Autodesk Fusion 360 part; units mm, degrees
(part 2 of 2)
  constraint coincident L135 L316.end
  constraint coincident L135 L317.end
  constraint coincident L135 L321.end
  constraint perpendicular L135 L321
  constraint coincident L135 L322.end
  constraint perpendicular L135 L322
  measures "d208" distance of L26.start L13.start
  measures "d209" distance of L9.start L13.start
  measures "d210" distance of L2.start L2.end
  measures "d211" distance of L1.start L2.end
  measures "d212" distance of L0.start L4.start
  measures "d213" distance of L23.start L21.end
  measures "d214" distance of L23.start L22.end
  measures "d217" distance of L8.start L54.end
  measures "d218" distance of L53.start L54.end
  measures "d234" distance of L40.start L40.end
  measures "d254" diameter of A0
  measures "d255" diameter of A2
  measures "d256" diameter of A12
  measures "d257" distance of L0.end L0.start
  measures "d265" distance of L10.start A1.centre
  measures "d266" distance of L10.start L10.end
  measures "d267" diameter of A3
  measures "d268" diameter of A1
  measures "d269" distance of L9.end L18.start
  measures "d270" distance of L9.end L17.start
  measures "d271" distance of L9.start L24.start
  measures "d272" distance of L9.start L11.start
  measures "d273" distance of L17.start L9.end
  measures "d274" distance of L11.start L28.start
  measures "d275" distance of L11.start L9.start
  measures "d276" distance of L38.start L18.end
  measures "d277" distance of L43.end L18.end
  measures "d278" diameter of A6
  measures "d279" distance of L35.start L24.end
  measures "d280" distance of L39.end L24.end
  measures "d281" diameter of A11
  measures "d300" distance of L22.start L63.end
  measures "d301" distance of L23.start L67.end
  measures "d303" distance of L71.start L71.end
  measures "d304" distance of L72.start L72.end
  measures "d305" distance of L55.end L73.end
  measures "d306" distance of L55.start L77.end
  measures "d307" distance of L57.end L84.end
  measures "d308" distance of L86.start L86.end
  measures "d310" distance of L5.start L91.end
  measures "d311" distance of L93.start L93.end
  measures "d312" distance of L94.start L94.end
  measures "d313" distance of L95.start L95.end
  measures "d314" distance of L96.start L96.end
  measures "d315" diameter of A13
  measures "d316" diameter of A14
  measures "d319" distance of L110.start L110.end
  measures "d320" distance of L110.start L111.end
  measures "d325" distance of L121.start L121.end
  measures "d326" distance of L121.start L122.end
  measures "d327" distance of L125.start L125.end
  measures "d328" distance of L125.start L129.end
  measures "d329" distance of L55.start L135.end
  measures "d334" distance of L0.end L139.end
  measures "d335" distance of L5.start L141.end
  measures "d336" distance of L4.start L145.end
  measures "d338" distance of L149.start L149.end
  measures "d339" distance of L149.start L150.end
  measures "d342" distance of L152.start L152.end
  measures "d343" distance of L152.start L153.end
  measures "d344" distance of L159.start L159.end
  measures "d345" distance of L159.start L160.end
  measures "d346" diameter of A15
  measures "d347" distance of L167.start L167.end
  measures "d348" distance of L168.start L168.end
  measures "d349" distance of L173.start L173.end
  measures "d350" distance of L174.start L174.end
  measures "d354" distance of L182.start L182.end
  measures "d356" distance of L188.start L188.end
  measures "d357" distance of L188.start L189.end
  measures "d358" distance of L194.start L194.end
  measures "d371" distance of L22.start L205.end
  measures "d372" distance of L22.end L209.end
  measures "d375" distance of L1.start L213.end
  measures "d376" distance of L2.end L217.end
  measures "d377" distance of L221.start L221.end
  measures "d378" distance of L222.start L222.end
  measures "d379" distance of L226.start L226.end
  measures "d380" distance of L1.end L231.end
  measures "d381" distance of L233.start L233.end
  measures "d382" distance of L233.start L236.end
  measures "d383" distance of L242.start L242.end
  measures "d384" distance of L242.start L243.end
  measures "d385" distance of L244.start L244.end
  measures "d386" distance of L244.start L245.end
  measures "d387" distance of L251.start L251.end
  measures "d388" distance of L251.start L252.end
  measures "d391" distance of L260.start L260.end
  measures "d392" distance of L260.start L262.end
  measures "d393" distance of L260.start L266.end
  measures "d396" distance of L270.start L270.end
  measures "d397" distance of L270.start L272.end
  measures "d398" distance of L270.start L270.end
  measures "d399" distance of L270.start L276.end
  measures "d400" diameter of A16
  measures "d401" diameter of A17
  measures "d404" distance of L13.start L290.end
  measures "d405" distance of L24.end L298.end
  measures "d411" distance of A8.centre L307.end
  measures "d412" distance of A4.centre L308.end
extrude "Extrude13" add sketch "v0.2" along normal blind 4 contours A0 L157 L164 | A0 L151 L157 L158 L164 A15 | A0 L157 L164 | A0 L157 L164 A15 | L158 L160 L164 A15 | L151 L152 L157 A15 | L5 L89 L158 L160 L161 | L0 L137 L149 L158 A15 | L0 L137 L149 L158 L159 L163 A15 | L5 L89 L151 L152 L154 | L0 L137 L150 L151 L153 L156 A15 | L0 L137 L150 L151 A15 | L146 L158 L159 L162 | L5 L16 L89 L90 L91 L145 | L0 L137 L149 L150 A15 | L0 L137 L138 L139 L140 L143 L147 L149 L150 A15 L233 L236 | L142 L151 L153 L155 | L5 L16 L89 L91 L92 L141 | L0 L4 L5 L89 L137 L145 L146 L147 L148 | L0 L5 L6 L89 L137 L141 L142 L143 L144 | L0 L137 L142 L150 L155 L156 | L31 L90 L91 L94 L99 L105 | L21 L91 L92 L95 L101 L116 | L31 L94 L96 L98 L104 L105 | L91 L166 L174 L176 | L23 L91 L165 L171 | L21 L93 L95 L97 L116 L117 | L23 L31 L67 L96 L102 L211 | L94 L99 L105 | L94 L98 A14 L105 | L23 L99 L166 L178 | L15 L23 L166 L175 | L23 L166 L174 L175 | L23 L165 L167 L171 | L23 L101 L165 L172 | L21 L23 L65 L93 L100 L207 | L95 A13 L116 | L95 L101 A13 L116 | L22 L23 L51 L67 L68 L69 L70 L209 L211 L212 | L23 L98 L102 L104 L108 | L98 A14 | L98 A14 L104 L105 | L15 L23 L166 L178 | L15 L22 L166 L175 L203 | L23 L165 L168 L172 | L10 L165 L167 L170 | L22 L23 L25 L63 L64 L65 L66 L205 L207 L208 | L23 L97 L100 L117 L119 | L95 L97 A13 | L95 L101 A13 | L97 A13 L116 L117 | L23 L68 L102 L210 L211 | L22 L62 L69 L72 L81 L209 | L98 A14 L109 | L23 A12 L98 A14 L107 | L10 L22 L165 L170 | L15 L166 L173 L178 | L10 L165 L168 L169 | L22 L61 L63 L86 L205 | L97 A13 L117 | A2 L23 L97 L101 A13 L118 | L101 A13 L120 | L23 L102 L210 | L22 L68 L81 L209 L210 | L62 L71 L72 L179 L180 | L23 A14 L104 | L23 L104 L108 | L23 A12 A14 L107 | L15 L178 L184 | L10 L22 L165 L169 | L22 L165 L170 L201 | L15 L22 L178 L181 L184 | L22 L166 L173 L177 | L22 L84 L166 L177 L204 | L22 L64 L87 L205 L206 | L22 L61 L84 L85 L86 L185 L186 | L23 A13 L117 | L23 L117 L119 | A2 L23 A13 L118 | L22 L81 L210 | L62 L71 L83 L84 L88 L179 | L22 L81 L112 L113 L180 | L23 A14 L104 L108 | L23 A12 A14 L107 | L15 L23 A12 A14 L107 | L10 L169 L193 | L10 L22 L169 L187 L193 | L22 L84 L165 L169 | L22 L177 L178 L181 L196 | L22 L177 L196 | L57 L75 L79 L82 L83 L84 L85 L127 L131 | A2 L10 L23 A13 L118 | L22 L86 L87 L206 | L55 L57 L58 L77 L78 L79 L80 L82 L133 | L22 L86 L185 | A2 L23 A13 L118 | L23 A13 L117 L119 | L55 L56 L57 L73 L74 L75 L76 L82 L133 | L88 L179 L181 L194 L195 | L15 A14 L199 | L15 A14 L103 L111 L199 | L22 L181 L182 L184 | L22 L169 L187 L192 | L22 L169 L192 | L22 L181 L194 L196 | L10 A13 L197 | L10 A13 L114 L121 L197 | L55 L73 L77 L125 L129 L133 L134 L135 L136 | L22 L103 L110 L111 L112 L113 | L179 L181 L182 L183 | L15 A14 L200 | L15 A14 | L22 L187 L189 L193 | L22 L187 L188 L192 | L10 A13 | L22 L114 L121 L122 L123 L124 | L55 L57 L82 L128 L129 L130 L131 L132 L133 | L22 L123 L124 L185 | L10 A13 L198 | L15 A14 L103 L110 L200 | L55 L57 L82 L125 L126 L127 L128 L132 L133 | L186 L187 L189 L190 | L186 L187 L188 L191 | L10 A13 L114 L122 L198 makes body 1
extrude "Extrude14" add sketch "v0.2" along normal blind 4 separate body contours L98 A14 L104 makes body 2
extrude "Extrude15" add sketch "v0.2" along normal blind 4 contours L15 L22 L166 L175 L203 bodies 1
combine "Combine1" operation add target body 1 tool bodies 2
extrude "Extrude16" add sketch "v0.2" along normal blind 4 contours L22 L166 L175 L201 L202 L203 L204 bodies 1
extrude "Extrude17" cut sketch "v0.2" along normal blind 4 contours L22 L170 L175 L202 bodies 1
extrude "Extrude18" add sketch "v0.2" along normal blind 4 contours L23 L64 L100 L206 L207 | L23 L100 L119 | L23 L100 L206 bodies 1
extrude "Extrude19" add sketch "v0.2" along normal blind 4 contours L15 L68 L102 L210 | L10 L64 L100 L206 | L15 L68 L81 L210 | L10 L64 L87 L206 bodies 1
copy_body "CopyPasteBodies1" bodies 1 makes body 3
extrude "Extrude20" add sketch "v0.2" along normal blind 4 contours L7 L138 L139 L222 L224 | L3 L139 L140 L226 L228 | L7 L221 L222 L223 | L3 L217 L218 L226 L227 | L7 L213 L214 L221 L225 | L2 L217 L218 L220 L239 | L1 L213 L214 L216 L239 | L224 L246 L247 L256 | L139 L233 L234 L236 L237 L258 | L2 L218 L220 L231 L239 | L228 L248 L249 L258 | L1 L214 L216 L231 L239 L250 L251 L252 | L214 L246 L256 L257 | L246 L247 L256 L257 | L234 L247 L256 L257 L258 L259 | L234 L237 L258 L259 | L2 L14 L218 L219 L220 L229 L230 L231 | L218 L249 L258 L259 | L248 L249 L258 L259 | L237 L248 L258 L259 | L1 L14 L214 L215 L216 L229 L231 L232 | L239 L246 L247 L255 L257 | L234 L262 L268 | L234 L237 L239 L259 L263 L273 | L9 L14 L19 L37 L44 L47 L214 L218 L229 L231 L235 L238 L240 L241 L242 L243 L244 L245 L292 | L218 L249 L253 L254 | L239 L248 L249 L259 | L239 L248 L249 L254 | L237 L272 L278 | L214 L231 L240 L246 L250 L253 | L214 L246 L250 L251 L252 L253 L254 | L239 L246 L247 L254 L255 | L234 L239 L260 L261 L262 L263 L264 A16 | L231 L241 L242 L243 L248 L249 L253 | L248 L249 L253 L254 | L237 L239 L270 L271 L272 L273 L274 A17 | L231 L240 L244 L245 L246 L247 L253 | L246 L247 L253 L254 | L234 L239 L260 L264 L265 L266 L267 A16 | L234 L237 L239 L254 L267 L277 | L234 L247 L253 L254 | L237 L248 L253 L254 | L237 L239 L270 L274 L275 L276 L277 A17 | L234 L266 L269 | L234 L237 L253 L254 | L237 L276 L279 | L231 L234 L235 L237 L238 L253 bodies 3
extrude "Extrude21" add sketch "v0.2" along normal blind 4 contours L9 L14 L17 L20 L27 L29 L37 L47 L229 L306 | L9 L11 L13 L14 L19 L28 L32 L44 L229 L305 | L9 L14 L18 L20 A5 L47 L229 L306 | L17 L20 L27 L29 L36 L49 L280 L306 | L9 L14 L24 L28 L44 A9 L229 L300 L305 | L11 L13 L28 L32 L33 L46 L284 L305 | L18 L20 L36 L38 L43 A5 A6 L297 L306 | L29 L36 L49 L280 L281 L283 L290 | L24 L28 L33 L35 L39 A9 A11 L299 L300 L305 | L13 L33 L46 L284 L285 L287 L290 | L26 L29 L281 L282 L283 L288 L289 L290 | L9 L14 L229 L295 L301 L303 L310 L312 | L33 L48 L287 L290 L295 L296 | L13 L26 L34 L41 L285 L286 L287 L288 L290 L291 | L9 L14 L229 L292 L293 L295 L301 | L18 L301 L302 L311 | L18 L36 L38 L43 A6 L45 L50 L297 | L26 L283 L288 L290 L293 | L24 L300 L303 L304 L312 | L24 L33 L35 L39 L42 L48 A11 L299 | L26 L287 L288 L290 L295 | L293 L295 L301 L302 | L293 L301 L302 L311 | L18 L302 L306 L311 | L18 L50 L293 L296 L297 L298 | L290 L293 L295 L296 | L26 L288 L290 L293 L294 L295 | L295 L301 L302 L303 L304 L312 | L24 L300 L304 L305 L312 | L24 L42 L295 L296 L298 L299 | L40 L293 L295 L302 L305 | L40 L293 L302 L305 L306 L311 | L293 L295 L296 L298 | L295 L302 L304 L305 L312 | L295 L298 L305 L312 | L40 L293 L295 L298 L305 bodies 3
extrude "Extrude22" add sketch "v0.2" along normal blind 4 contours L9 L14 L18 L229 L307 L309 | L9 L14 L24 L229 L300 L308 L310 | L18 L301 L307 L311 | L24 L300 L303 L308 L312 | L18 L298 L306 L311 | L24 L298 L300 L305 L312 bodies 3
extrude "Extrude23" cut sketch "v0.2" along normal blind 4 contours L40 L293 L295 L302 L305 | L40 L293 L302 L305 L306 L311 | L295 L302 L304 L305 L312 bodies 3
extrude "Extrude24" add sketch "v0.2" along normal blind 4 contours L40 L293 L295 L302 L305 bodies 3
extrude "Extrude25" add sketch "v0.2" along normal blind 4 contours L8 L12 L53 L54 L59 L60 L134 L135 L136 L313 L314 L315 L316 L317 L318 L319 L320 L321 L322 | L135 L313 L314 L317 L318 L321 | L135 L315 L316 L319 L320 L322 | L135 L313 L315 L321 L322 | L313 L315 L321 | L313 L315 L322 bodies 3
extrude "Extrude26" cut sketch "v0.2" along normal blind 4 contours L135 L313 L314 L317 L318 L321 | L135 L315 L316 L319 L320 L322 bodies 3
extrude "Extrude27" cut sketch "v0.2" along normal blind 4 contours A0 L157 L164 | A0 L157 L164 | L0 L137 L142 L150 L155 L156 | L214 L231 L240 L246 L250 L253 | L9 L14 L229 L295 L301 L303 L310 L312 | L33 L48 L287 L290 L295 L296 | L295 L298 L305 L312 bodies 3
extrude "Extrude2" [suppressed]
extrude "Extrude3" [suppressed]
hidden bodies 1
equation "d108 = ( 104 / 2 ) * 1 mm"
equation "d109 = ( 104 / 2 ) * 1 mm"
equation "d265 = ( 104 / 2 ) * 1 mm"
equation "d266 = ( 104 / 2 ) * 1 mm"
named bodies: "CarBodyRearEnd"
